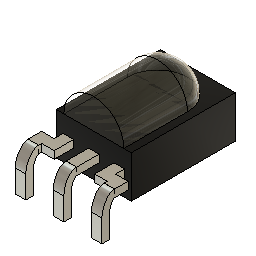
IRIO3 (Autodesk Fusion 360 archive; units mm, degrees)
design "TSOP"
Autodesk Fusion 360 part; units mm, degrees
sketch "Sketch2" plane through (0, 0, 0) normal (0, 0, 1) x (1, 0, 0)
  line L0 (4, 1) -> (-4, 1) construction
  line L1 (-4, 1) -> (-4, -1) construction
  line L2 (-4, -1) -> (4, -1) construction
  line L3 (4, -1) -> (4, 1) construction
  line L4 (4, 1) -> (-4, -1) construction
  line L5 (-4, 1) -> (4, -1) construction
  line L6 (0.35, -0.75) -> (-0.35, -0.75)
  line L7 (-0.35, -0.75) -> (-0.35, -1.25)
  line L8 (-0.35, -1.25) -> (0.35, -1.25)
  line L9 (0.35, -1.25) -> (0.35, -0.75)
  line L10 (0.35, -0.75) -> (-0.35, -1.25) construction
  line L11 (-0.35, -0.75) -> (0.35, -1.25) construction
  line L12 (2.89, -0.75) -> (2.19, -0.75)
  line L13 (2.19, -0.75) -> (2.19, -1.25)
  line L14 (2.19, -1.25) -> (2.89, -1.25)
  line L15 (2.89, -1.25) -> (2.89, -0.75)
  line L16 (2.89, -0.75) -> (2.19, -1.25) construction
  line L17 (2.19, -0.75) -> (2.89, -1.25) construction
  line L18 (0, -1) -> (0, -1.849) construction
  line L19 (-2.89, -0.75) -> (-2.19, -0.75)
  line L20 (-2.89, -1.25) -> (-2.89, -0.75)
  line L21 (-2.19, -0.75) -> (-2.89, -1.25) construction
  line L22 (-2.19, -0.75) -> (-2.19, -1.25)
  line L23 (-2.89, -0.75) -> (-2.19, -1.25) construction
  line L24 (-2.19, -1.25) -> (-2.89, -1.25)
  point P0 (0, -1)
  point P1 (2.54, -1)
  point P2 (-2.54, -1)
  dimension "d92" = 2
  dimension "d93" = 8
  dimension "d117" = 0.7
  dimension "d118" = 0.5
  dimension "d119" = 0.7
  dimension "d120" = 0.5
  dimension "d121" = 2.54
  constraint perpendicular L0 L1
  constraint parallel L0 L2
  constraint parallel L1 L3
  constraint horizontal L0
  constraint coincident L4 origin
  constraint coincident L5 origin
  constraint perpendicular L6 L7
  constraint parallel L6 L8
  constraint parallel L7 L9
  constraint horizontal L6
  constraint coincident L10 P0
  constraint coincident L11 P0
  constraint midpoint L2 P0
  constraint perpendicular L12 L13
  constraint parallel L12 L14
  constraint parallel L13 L15
  constraint horizontal L12
  constraint coincident L16 P1
  constraint coincident L17 P1
  constraint coincident L2 P1
  constraint coincident P0 L18.start
  constraint perpendicular L2 L18
  constraint symmetric L12.start L18 L19.start
  constraint symmetric L12.end L18 L19.end
  constraint symmetric L13.end L18 L22.end
  constraint symmetric L14.end L18 L20.start
  constraint symmetric P1 L18 P2
  measures "d92" distance of L0.end L1.end
  measures "d93" distance of L1.end L2.end
  measures "d117" distance of L7.end L8.end
  measures "d118" distance of L6.end L7.end
  measures "d119" distance of L13.end L14.end
  measures "d120" distance of L12.end L13.end
  measures "d121" distance of P0 P1
ref_plane "WorkPlane1" through (0, 1, 0) normal (0, 1, 0) x (-1, 0, 0) in component "Case"
sketch "Sketch1" plane through (0, 1, 0) normal (0, 1, 0) x (-1, 0, 0) in component "Case"
  line L0 (0, 0) -> (0, 2) construction
  line L1 (2.5, 0.6) -> (-2.5, 0.6)
  line L2 (-2.5, 0.6) -> (-2.5, 3.4)
  line L3 (-2.5, 3.4) -> (2.5, 3.4)
  line L4 (2.5, 3.4) -> (2.5, 0.6)
  line L5 (2.5, 0.6) -> (-2.5, 3.4) construction
  line L6 (-2.5, 0.6) -> (2.5, 3.4) construction
  point P0 (0, 2)
  dimension "d95" = 2
  dimension "d96" = 5
  dimension "d97" = 2.8
  constraint coincident L0.start origin
  constraint perpendicular L1 L2
  constraint parallel L1 L3
  constraint parallel L2 L4
  constraint horizontal L1
  constraint coincident L5 P0
  constraint coincident L6 P0
  constraint coincident P0 L0.end
  constraint vertical L0
  measures "d95" distance of L0.start P0
  measures "d96" distance of L2.end L3.end
  measures "d97" distance of L1.end L2.end
extrude "Extrude2" add sketch "Sketch1" along normal blind 6.95 from surface at 0.1 makes body 1 in component "Case"
sketch "Sketch2 (2)" plane through (0, 1.1, 0) normal (0, -1, 0) x (1, 0, 0) in component "Lens"
  line L0 (2.5, 3.4) -> (-2.5, 3.4)
  line L1 (-2.5, 3.4) -> (-2.5, 0.6)
  line L2 (-2.5, 0.6) -> (2.5, 0.6)
  line L3 (2.5, 0.6) -> (2.5, 3.4)
  circle A0 centre (0, 3.4) radius 2
  dimension "d100" = 4
  constraint midpoint L0 A0.centre
  measures "d100" diameter of A0
extrude "Extrude3" add sketch "Sketch2 (2)" against normal blind 6.25 separate body contours L0 A0 picked at (0.4157, 3.9212) makes body 2 in component "Lens"
fillet "Fillet2" radius 2 1 edges at (0, 7.35, 5.4) on bodies 2 in component "Lens"
ref_plane "WorkPlane1" through (0, 4.575, 2) normal (0, 0, 1) x (1, 0, 0) in component "Leads"
sketch "zigzag" plane through (0, 7.975, 2) normal (0, 0, 1) x (1, 0, 0) in component "Leads"
  line L0 (-2.5, -6.875) -> (2.5, -6.875)
  line L1 (2.5, -6.875) -> (2.5, 0.075) construction
  line L2 (2.5, 0.075) -> (-2.5, 0.075) construction
  line L3 (-2.5, 0.075) -> (-2.5, -6.875) construction
  line L4 (0, -6.875) -> (0, -11.875) construction
  line L5 (0.35, -6.875) -> (-0.35, -6.875)
  line L6 (-0.35, -6.875) -> (-0.35, -8.375)
  line L7 (-0.35, -8.375) -> (0.35, -8.375)
  line L8 (0.35, -8.375) -> (0.35, -6.875)
  line L9 (0.35, -6.875) -> (-0.35, -8.375) construction
  line L10 (-0.35, -6.875) -> (0.35, -8.375) construction
  line L11 (2.89, -8.375) -> (2.19, -8.375)
  line L12 (2.19, -8.375) -> (2.19, -8.175)
  line L13 (2.19, -8.175) -> (2.89, -8.175)
  line L14 (2.89, -8.175) -> (2.89, -8.375)
  line L15 (2.89, -8.375) -> (2.19, -8.175) construction
  line L16 (2.19, -8.375) -> (2.89, -8.175) construction
  line L17 (2.89, -8.175) -> (2.89, -7.475)
  line L18 (2.89, -7.475) -> (2.05, -7.475)
  line L19 (2.05, -7.475) -> (2.05, -6.875)
  line L20 (1.35, -6.875) -> (1.35, -8.175)
  line L21 (1.35, -8.175) -> (2.19, -8.175)
  line L22 (-2.19, -8.175) -> (-2.89, -8.175)
  line L23 (-2.89, -7.475) -> (-2.05, -7.475)
  line L24 (-1.35, -6.875) -> (-1.35, -8.175)
  line L25 (-2.89, -8.375) -> (-2.19, -8.375)
  line L26 (-2.19, -8.375) -> (-2.89, -8.175) construction
  line L27 (-2.19, -8.375) -> (-2.19, -8.175)
  line L28 (-2.05, -7.475) -> (-2.05, -6.875)
  line L29 (-1.35, -8.175) -> (-2.19, -8.175)
  line L30 (-2.89, -8.175) -> (-2.89, -8.375)
  line L31 (-2.89, -8.375) -> (-2.19, -8.175) construction
  line L32 (-2.89, -8.175) -> (-2.89, -7.475)
  point P0 (0, -7.625)
  point P1 (2.54, -8.275)
  point P2 (-2.5, -6.875)
  point P3 (-2.54, -8.275)
  dimension "d104" = 5
  dimension "d105" = 0.7
  dimension "d106" = 1.5
  dimension "d107" = 0.7
  dimension "d109" = 2.54
  dimension "d110" = 0.7
  dimension "d111" = 0.7
  dimension "d112" = 1.54
  dimension "d113" = 1.3
  constraint midpoint L0 L4.start
  constraint perpendicular L0 L4
  constraint perpendicular L5 L6
  constraint parallel L5 L7
  constraint parallel L6 L8
  constraint horizontal L5
  constraint coincident L9 P0
  constraint coincident L10 P0
  constraint coincident L4 P0
  constraint collinear L0 L5
  constraint perpendicular L11 L12
  constraint parallel L11 L13
  constraint parallel L12 L14
  constraint horizontal L11
  constraint coincident L15 P1
  constraint coincident L16 P1
  constraint collinear L7 L11
  constraint perpendicular L13 L17
  constraint perpendicular L17 L18
  constraint coincident L0 L19.end
  constraint perpendicular L0 L19
  constraint coincident L0 L20.start
  constraint perpendicular L0 L20
  constraint perpendicular L20 L21
  constraint symmetric L0.end L4 L0.start
  constraint symmetric L4 L11.start L25.start
  constraint symmetric L4 L11.end L25.end
  constraint symmetric L4 L12.end L22.start
  constraint symmetric L4 L13.end L22.end
  constraint symmetric L4 P1 P3
  constraint symmetric L4 L17.end L23.start
  constraint symmetric L4 L18.end L23.end
  constraint symmetric L4 L19.end L28.end
  constraint symmetric L4 L20.start L24.start
  constraint symmetric L4 L20.end L24.end
  measures "d104" distance of L4.start L4.end
  measures "d105" distance of L6.end L7.end
  measures "d106" distance of L5.end L6.end
  measures "d107" distance of L12.end L13.end
  measures "d109" distance of L4 P1
  measures "d110" distance of L18 L21
  measures "d111" distance of L19 L20
  measures "d112" distance of L14 L20
  measures "d113" distance of L20.start L20.end
extrude "Extrude2'" add sketch "zigzag" along normal mid plane 0.5 separate body makes body 3 at (-1.5833, 0.4667, 2.25) makes body 4 at (0.1167, 0.6, 2.25) makes body 5 at (1.5833, 0.4667, 2.25) in component "Leads"
sketch "zigzag base" plane through (0, -0.4, 0) normal (0, -1, 0) x (1, 0, 0) in component "Leads"
  line L0 (0.35, 1.75) -> (0.35, 2.25) construction
  line L1 (0.35, 2.25) -> (-0.35, 2.25) construction
  line L2 (-0.35, 2.25) -> (-0.35, 1.75) construction
  line L3 (-0.35, 1.75) -> (0.35, 1.75) construction
  line L4 (-2.19, 1.75) -> (-2.19, 2.25) construction
  line L5 (-2.19, 2.25) -> (-2.89, 2.25) construction
  line L6 (-2.89, 2.25) -> (-2.89, 1.75) construction
  line L7 (-2.89, 1.75) -> (-2.19, 1.75) construction
  line L8 (2.89, 1.75) -> (2.89, 2.25) construction
  line L9 (2.89, 2.25) -> (2.19, 2.25) construction
  line L10 (2.19, 2.25) -> (2.19, 1.75) construction
  line L11 (2.19, 1.75) -> (2.89, 1.75) construction
  line L12 (-2.89, 2) -> (2.9, 2) construction
  line L13 (-2.54, 2.25) -> (-2.54, 1.75) construction
  line L14 (0, 2.25) -> (0, 1.75) construction
  line L15 (2.54, 2.25) -> (2.54, 1.75) construction
  circle A0 centre (-2.54, 2) radius 0.25
  circle A1 centre (2.54, 2) radius 0.25
  circle A2 centre (0, 2) radius 0.25
  dimension "d124" = 0.5
  dimension "d126" = 0.5
  dimension "d127" = 0.5
  constraint midpoint L6 L12.start
  constraint perpendicular L10 L12
  constraint midpoint L5 L13.start
  constraint midpoint L7 L13.end
  constraint midpoint L1 L14.start
  constraint midpoint L3 L14.end
  constraint midpoint L9 L15.start
  constraint midpoint L11 L15.end
  constraint midpoint L13 A0.centre
  constraint midpoint L15 A1.centre
  constraint midpoint L14 A2.centre
  measures "d124" diameter of A0
  measures "d126" diameter of A1
  measures "d127" diameter of A2
extrude "Extrude3'" add sketch "Sketch2" along normal blind 1 and the other way blind 0.5 separate body makes body 6 at (-2.4233, -1.25, 0) makes body 7 at (-0.1167, -1.25, 0) makes body 8 at (2.4233, -1.25, 0) in component "Leads"
sketch "base top" plane through (0, 0, 1) normal (0, 0, 1) x (-1, 0, 0) in component "Leads"
  line L0 (-0.35, 1.25) -> (-0.35, 0.75)
  line L1 (-0.35, 0.75) -> (0.35, 0.75)
  line L2 (0.35, 0.75) -> (0.35, 1.25)
  line L3 (0.35, 1.25) -> (-0.35, 1.25)
  line L4 (2.89, 0.75) -> (2.19, 0.75) construction
  line L5 (2.89, 1.25) -> (2.89, 0.75) construction
  line L6 (2.19, 1.25) -> (2.89, 1.25) construction
  line L7 (2.19, 0.75) -> (2.19, 1.25) construction
  line L8 (-0.35, 0.75) -> (0.35, 0.75) construction
  line L9 (0.35, 0.75) -> (0.35, 1.25) construction
  line L10 (0.35, 1.25) -> (-0.35, 1.25) construction
  line L11 (-0.35, 1.25) -> (-0.35, 0.75) construction
  line L12 (-2.89, 0.75) -> (-2.19, 0.75) construction
  line L13 (-2.19, 0.75) -> (-2.19, 1.25) construction
  line L14 (-2.89, 1.25) -> (-2.89, 0.75) construction
  line L15 (-2.19, 1.25) -> (-2.89, 1.25) construction
  spline S0 degree 5 poles (2.54, 1, 0) (2.54, 1.003, 0.069) (2.54, 0.9992, 0.2017) (2.54, 0.9642, 0.3851) (2.54, 0.8688, 0.5999) (2.54, 0.7062, 0.8167) (2.54, 0.5711, 0.9371) (2.54, 0.4799, 0.9866) (2.54, 0.4256, 0.999) (2.54, 0.4, 1) knots 0 0 0 0 0 0 0.2 0.4 0.6 0.8 1 1 1 1 1 1
  spline S1 degree 5 poles (0, 1, 0) (0, 0.9998, 0.0673) (0, 0.9927, 0.1973) (0, 0.9615, 0.3785) (0, 0.8848, 0.5935) (0, 0.7488, 0.813) (0, 0.6191, 0.9358) (0, 0.5129, 0.9864) (0, 0.4383, 0.999) (0, 0.4, 1) knots 0 0 0 0 0 0 0.2 0.4 0.6 0.8 1 1 1 1 1 1
  spline S2 degree 5 poles (-2.54, 1, 0) (-2.54, 0.999, 0.054) (-2.54, 0.9907, 0.1624) (-2.54, 0.9598, 0.326) (-2.54, 0.8862, 0.5423) (-2.54, 0.7552, 0.7848) (-2.54, 0.6269, 0.927) (-2.54, 0.5184, 0.9855) (-2.54, 0.4404, 0.9994) (-2.54, 0.4, 1) knots 0 0 0 0 0 0 0.2 0.4 0.6 0.8 1 1 1 1 1 1
  line L16 (-2.54, 0.7991, 0.9939) -> (-2.54, 0.0009, 1.0061)
  line L17 (-2.54, 1.0117, -0.6181) -> (-2.54, 0.9883, 0.6181)
  line L18 (0, 0.552, 0.996) -> (0, 0.248, 1.004)
  line L19 (0, 1.0008, -0.3075) -> (0, 0.9992, 0.3075)
  line L20 (2.54, 0.502, 0.996) -> (2.54, 0.298, 1.004)
  line L21 (2.54, 0.9865, -0.3115) -> (2.54, 1.0135, 0.3115)
  point P0 (2.54, 1)
  point P1 (0, 1)
  point P2 (-2.54, 1)
  point P3 (2.54, 0.4)
  point P4 (0, 0.4)
  point P5 (-2.54, 0.4)
sweep "Sweep5" add profiles "base top" path "base top" along S1 section 1 bodies 4 7 in component "Leads"
sweep "Sweep4" add 1 faces at (2.6567, -1.0833, 1) path "base top" along S2 on bodies 8 bodies 8 5 in component "Leads"
sweep "Sweep6" add 1 faces at (-2.4233, -1.0833, 1) path "base top" along S0 on bodies 6 bodies 6 3 in component "Leads"
component "Case" placed x (1, 0, 0) y (0, 1, 0) z (0, 0, 1) at (0, 0, 0)
component "Lens" placed x (1, 0, 0) y (0, 1, 0) z (0, 0, 1) at (0, 0, 0)
component "Leads" placed x (1, 0, 0) y (0, 1, 0) z (0, 0, 1) at (0, 0, 0)
equation "Height = 0.1 mm"
equation "BendAngle = 90 deg"
equation "Hinge = 2 mm"
equation "d92 = Hinge"
equation "d94 = BendAngle"
equation "d95 = Hinge"
equation "d113 = 8.25 mm - 6.95 mm"
equation "d116 = Height"
named bodies: "GND", "Signal", "V+"

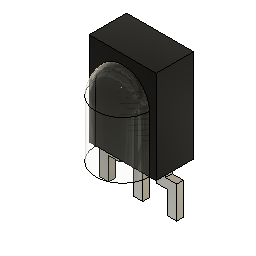
design "TSOP (Straight)"
Autodesk Fusion 360 part; units mm, degrees
sketch "Sketch2" plane through (0, 0, 0) normal (0, 0, 1) x (1, 0, 0) in component "Case"
  line L0 (2.5, -1.4) -> (-2.5, -1.4)
  line L1 (-2.5, -1.4) -> (-2.5, 1.4)
  line L2 (-2.5, 1.4) -> (2.5, 1.4)
  line L3 (2.5, 1.4) -> (2.5, -1.4)
  line L4 (2.5, -1.4) -> (-2.5, 1.4) construction
  line L5 (-2.5, -1.4) -> (2.5, 1.4) construction
  dimension "d148" = 5
  dimension "d149" = 2.8
  constraint perpendicular L0 L1
  constraint parallel L0 L2
  constraint parallel L1 L3
  constraint horizontal L0
  constraint coincident L4 origin
  constraint coincident L5 origin
  measures "d148" distance of L1.end L2.end
  measures "d149" distance of L0.end L1.end
extrude "Extrude2" add sketch "Sketch2" along normal blind 6.95 from surface at 5 makes body 1 in component "Case"
sketch "Sketch2 (2)" plane through (0, 0, 5) normal (0, 0, -1) x (1, 0, 0) in component "Lens"
  circle A0 centre (0, 1.4) radius 2
  line L0 (-2.5, -1.4) -> (2.5, -1.4)
  line L1 (2.5, -1.4) -> (2.5, 1.4)
  line L2 (2.5, 1.4) -> (-2.5, 1.4)
  line L3 (-2.5, 1.4) -> (-2.5, -1.4)
  dimension "d100" = 4
  measures "d100" diameter of A0
extrude "Extrude3" add sketch "Sketch2 (2)" against normal blind 6.25 separate body contours A0 L2 picked at (0.5508, 1.7755) makes body 2 in component "Lens"
fillet "Fillet2" radius 2 1 edges at (0, -3.4, 11.25) on bodies 2 in component "Lens"
sketch "zigzag" plane through (0, 0, 8.475) normal (0, 1, 0) x (1, 0, 0) in component "Leads"
  line L0 (-2.5, 3.475) -> (2.5, 3.475) construction
  line L1 (2.5, 3.475) -> (2.5, -3.475) construction
  line L2 (2.5, -3.475) -> (-2.5, -3.475) construction
  line L3 (-2.5, -3.475) -> (-2.5, 3.475) construction
  line L4 (1.35, 3.475) -> (1.35, 4.775)
  line L5 (1.35, 4.775) -> (2.19, 4.775)
  line L6 (2.19, 4.775) -> (2.19, 6.475)
  line L7 (2.19, 6.475) -> (2.89, 6.475)
  line L8 (2.89, 6.475) -> (2.89, 4.075)
  line L9 (2.89, 4.075) -> (2.05, 4.075)
  line L10 (2.05, 4.075) -> (2.05, 3.5)
  line L11 (2.05, 3.5) -> (1.35, 3.475)
  line L12 (0, 3.475) -> (0, 11.475) construction
  line L13 (-0.35, 3.475) -> (0.35, 3.475)
  line L14 (0.35, 3.475) -> (0.35, 6.475)
  line L15 (0.35, 6.475) -> (-0.35, 6.475)
  line L16 (-0.35, 6.475) -> (-0.35, 3.475)
  line L17 (-0.35, 3.475) -> (0.35, 6.475) construction
  line L18 (0.35, 3.475) -> (-0.35, 6.475) construction
  line L19 (2.54, 6.475) -> (2.54, 5.7) construction
  line L20 (-2.54, 6.475) -> (-2.54, 5.7) construction
  line L21 (-1.35, 3.475) -> (-1.35, 4.775)
  line L22 (-2.89, 4.075) -> (-2.05, 4.075)
  line L23 (-2.05, 3.5) -> (-1.35, 3.475)
  line L24 (-1.35, 4.775) -> (-2.19, 4.775)
  line L25 (-2.19, 4.775) -> (-2.19, 6.475)
  line L26 (-2.19, 6.475) -> (-2.89, 6.475)
  line L27 (-2.05, 4.075) -> (-2.05, 3.5)
  line L28 (-2.89, 6.475) -> (-2.89, 4.075)
  point P0 (0, 4.975)
  point P1 (-2.5, 3.475)
  dimension "d49" = 0
  dimension "d50" = 0
  dimension "d51" = 0
  dimension "d52" = 0
  dimension "d72" = 0
  dimension "d73" = 0
  dimension "d74" = 0
  dimension "d75" = 0
  dimension "d152" = 0.7
  dimension "d153" = 0.7
  dimension "d154" = 1.3
  dimension "d155" = 0.7
  dimension "d156" = 8
  dimension "d157" = 3
  dimension "d158" = 0.7
  dimension "d159" = 1.54
  dimension "d160" = 2.54
  constraint coincident L0 L4.start
  constraint perpendicular L0 L4
  constraint perpendicular L4 L5
  constraint perpendicular L0 L6
  constraint perpendicular L4 L7
  constraint perpendicular L7 L8
  constraint perpendicular L8 L9
  constraint perpendicular L9 L10
  constraint midpoint L0 L12.start
  constraint perpendicular L0 L12
  constraint perpendicular L13 L14
  constraint parallel L13 L15
  constraint parallel L14 L16
  constraint horizontal L13
  constraint coincident L17 P0
  constraint coincident L18 P0
  constraint coincident L12 P0
  constraint collinear L0 L13
  constraint collinear L7 L15
  constraint midpoint L7 L19.start
  constraint perpendicular L7 L19
  constraint symmetric L0.end L12 P1
  constraint symmetric L4.start L12 L21.start
  constraint symmetric L4.end L12 L21.end
  constraint symmetric L5.end L12 L24.end
  constraint symmetric L6.end L12 L25.end
  constraint symmetric L7.end L12 L26.end
  constraint symmetric L8.end L12 L22.start
  constraint symmetric L9.end L12 L22.end
  constraint symmetric L10.end L12 L23.start
  constraint symmetric L12 L19.start L20.start
  constraint symmetric L12 L19.end L20.end
  measures "d152" distance of L6.end L7.end
  measures "d153" horizontal distance of L4.start L10.end
  measures "d154" distance of L4.start L4.end
  measures "d155" distance of L5.end L9
  measures "d156" distance of L12.start L12.end
  measures "d157" distance of L13.end L14.end
  measures "d158" distance of L14.end L15.end
  measures "d159" distance of L4 L8
  measures "d160" distance of L12 L19
extrude "Extrude2'" add sketch "zigzag" along normal mid plane 0.5 separate body makes body 3 at (-2.6567, 0.25, 3.3667) makes body 4 at (2.6567, 0.25, 3.3667) makes body 5 at (0.1167, 0.25, 3) in component "Leads"
component "Case" placed x (1, 0, 0) y (0, 1, 0) z (0, 0, 1) at (0, 0, 0)
component "Lens" placed x (1, 0, 0) y (0, 1, 0) z (0, 0, 1) at (0, 0, 0)
component "Leads" placed x (1, 0, 0) y (0, 1, 0) z (0, 0, 1) at (0, 0, 0)
equation "Height = 5 mm"
equation "d116 = Height"
equation "d157 = LeadLenght"
equation "LeadLenght = 3 mm"
equation "d113 = 8.25 mm - 6.95 mm"
named bodies: "Signal", "+V", "GND"
